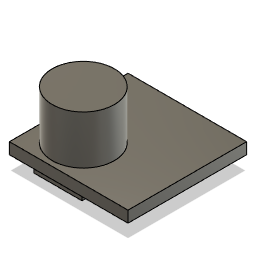
smallRegulator (Autodesk Fusion 360 design; units mm, degrees)
Autodesk Fusion 360 part; units mm, degrees
sketch "Sketch1" plane through (0, 0, 0) normal (0, 1, 0) x (1, 0, 0)
  line L0 (0, 0) -> (10.5, 0)
  line L1 (10.5, 0) -> (10.5, 10.5)
  line L2 (10.5, 10.5) -> (0, 10.5)
  line L3 (0, 10.5) -> (0, 0)
  dimension "d1" = 10.5
  dimension "d2" = 10.5
  constraint horizontal L0
  constraint vertical L1
  constraint horizontal L2
  constraint vertical L3
  constraint coincident L0.start L3.end
  measures "d1" distance of L0.start L0.end
  measures "d2" distance of L0.start L2.end
extrude "Extrude1" add sketch "Sketch1" along normal blind 1
sketch "Sketch2" plane through (0, 1, 0) normal (0, 1, 0) x (-1, 0, 0)
  line L0 (0, -10.5) -> (0, 0)
  line L1 (0, 0) -> (-10.5, 0)
  line L2 (-10.5, 0) -> (-10.5, -10.5)
  line L3 (-10.5, -10.5) -> (0, -10.5)
  circle A0 centre (-3.3528, -3.1902) radius 2.75
  dimension "d5" = 5.5
  measures "d5" diameter of A0
extrude "Extrude2" add sketch "Sketch2" along normal blind 4.3 contours A0
sketch "Sketch3" plane through (0, 0, 0) normal (0, -1, 0) x (1, 0, 0)
  line L0 (0, 0) -> (0, -10.5)
  line L1 (0, -10.5) -> (10.5, -10.5)
  line L2 (10.5, -10.5) -> (10.5, 0)
  line L3 (10.5, 0) -> (0, 0)
  line L4 (1.2846, -0.8796) -> (5.5502, -0.8796)
  line L5 (5.5502, -0.8796) -> (5.5502, -9.7985)
  line L6 (5.5502, -9.7985) -> (1.2846, -9.7985)
  line L7 (1.2846, -9.7985) -> (1.2846, -0.8796)
  constraint horizontal L4
  constraint vertical L5
  constraint horizontal L6
  constraint vertical L7
extrude "Extrude3" add sketch "Sketch3" along normal blind 1.2 contours L4 L5 L6 L7
